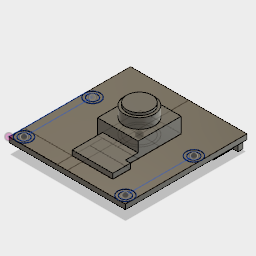
Pi Camera v2 (Autodesk Fusion 360 design; units mm, degrees)
Autodesk Fusion 360 part; units mm, degrees
sketch "Sketch1" plane through (0, 0, 0) normal (0, 1, 0) x (1, 0, 0)
  line L0 (0, 0) -> (23, 0)
  line L1 (23, 0) -> (23, 24)
  line L2 (23, 24) -> (0, 24)
  line L3 (0, 24) -> (0, 0)
  line L4 (0, 0) -> (9.4996, 0)
  line L5 (0, 3.5052) -> (0, 0)
  line L6 (0, 0) -> (9.5, 0)
  line L7 (0, 3) -> (0, 0)
  line L8 (9.5, 3) -> (17.5, 3)
  line L9 (17.5, 3) -> (17.5, 6.5)
  line L10 (17.5, 6.5) -> (9.5, 6.5)
  line L11 (9.5, 6.5) -> (9.5, 3)
  line L12 (9.5, 3) -> (0, 3)
  line L13 (9.5, 6.5) -> (16.5, 6.5)
  line L14 (16.5, 6.5) -> (16.5, 9)
  line L15 (16.5, 9) -> (9.5, 9)
  line L16 (9.5, 9) -> (9.5, 6.5)
  line L17 (16.5, 9) -> (7.5, 9)
  line L18 (7.5, 9) -> (7.5, 17.5)
  line L19 (7.5, 17.5) -> (16.5, 17.5)
  line L20 (16.5, 17.5) -> (16.5, 9)
  line L21 (12, 17.5) -> (12, 9)
  line L22 (7.5, 13.25) -> (16.5, 13.25)
  circle A0 centre (12, 13.25) radius 3.25
  circle A1 centre (12, 13.25) radius 2.5
  dimension "d1" = 23
  dimension "d2" = 24
  dimension "d22" = 9.5
  dimension "d23" = 3
  dimension "d25" = 3.5
  dimension "d28" = 7
  dimension "d29" = 2.5
  dimension "d30" = 8.5
  dimension "d31" = 9
  dimension "d32" = 6.5
  dimension "d33" = 5
  measures "d1" distance of L0.start L0.end
  measures "d2" distance of L0.start L2.end
  measures "d22" distance of L0.start L6.end
  measures "d23" distance of L0.start L7.start
  measures "d25" distance of L8.start L10.end
  measures "d28" distance of L10.end L13.end
  measures "d29" distance of L10.end L15.end
  measures "d30" distance of L14.end L19.end
  measures "d31" distance of L14.end L17.end
  measures "d32" diameter of A0
  measures "d33" diameter of A1
extrude "Extrude4" add sketch "Sketch1" along normal blind 1 contours L0 L1 L2 L3 L4 L5 L6 L7 | L8 L9 L10 L11 L13 | L10 L13 L14 L15 L16 L17 | L15 L17 L18 L21 L22 A0 | L15 L17 L20 L21 L22 A0 | L19 L20 L21 L22 A0 | L21 L22 A0 A1 | L21 L22 A0 A1 | L18 L19 L21 L22 A0 | L21 L22 A0 A1 | L21 L22 A1 | L21 L22 A1 | L21 L22 A0 A1 | L21 L22 A1 | L21 L22 A1 makes body 1
extrude "Extrude1" add sketch "Sketch1" along normal blind 1 separate body contours L0 L1 L2 L3 L4 L5 L6 L7 | L8 L9 L10 L11 L13 | L10 L13 L14 L15 L16 L17 | L15 L17 L18 L21 L22 A0 | L15 L17 L20 L21 L22 A0 | L19 L20 L21 L22 A0 | L21 L22 A0 A1 | L21 L22 A0 A1 | L18 L19 L21 L22 A0 | L21 L22 A0 A1 | L21 L22 A1 | L21 L22 A1 | L21 L22 A0 A1 | L21 L22 A1 | L21 L22 A1 makes body 2
sketch "Sketch2" plane through (0, 1, 0) normal (0, 1, 0) x (-1, 0, 0)
  line L0 (0, -24) -> (0, 0)
  line L1 (0, 0) -> (-23, 0)
  line L2 (-23, 0) -> (-23, -24)
  line L3 (-23, -24) -> (0, -24)
  line L4 (0, 0) -> (-9.5, 0)
  line L5 (-9.5, 0) -> (-9.5, -3)
  line L6 (-9.5, -3) -> (0, -3)
  line L7 (0, -3) -> (0, 0)
  line L8 (-9.5, -3) -> (-17.5, -3)
  line L9 (-17.5, -3) -> (-17.5, -6.5)
  line L10 (-17.5, -6.5) -> (-9.5, -6.5)
  line L11 (-9.5, -6.5) -> (-9.5, -3)
  line L12 (-9.5, -6.5) -> (-16.5, -6.5)
  line L13 (-16.5, -6.5) -> (-16.5, -9)
  line L14 (-16.5, -9) -> (-9.5, -9)
  line L15 (-9.5, -9) -> (-9.5, -6.5)
  line L16 (-16.5, -9) -> (-8.5, -9)
  line L17 (-8.5, -9) -> (-8.5, -17.5)
  line L18 (-8.5, -17.5) -> (-16.5, -17.5)
  line L19 (-16.5, -17.5) -> (-16.5, -9)
  line L20 (-12.5, -17.5) -> (-12.5, -9)
  line L21 (-8.5, -13.25) -> (-16.5, -13.25)
  circle A0 centre (-12.5, -13.25) radius 3
  circle A1 centre (-12.5, -13.25) radius 2.5
  line L22 (0, 0) -> (0, -15)
  line L23 (0, -15) -> (-1.5, -15)
  circle A2 centre (-1.5, -15) radius 1.5
  line L24 (-11.5, -24) -> (-11.5, 0)
  circle A3 centre (-21.5, -15) radius 1.5
  line L25 (-1.5, -15) -> (-1.5, -1.5)
  circle A4 centre (-1.5, -1.5) radius 1.4986
  line L26 (-21.5, -15) -> (-21.5, -1.5)
  circle A5 centre (-21.5, -1.5) radius 1.4986
  circle A6 centre (-1.5, -15) radius 1
  circle A7 centre (-1.5, -1.5) radius 1
  circle A8 centre (-21.5, -1.5) radius 1
  circle A9 centre (-21.5, -15) radius 1
  dimension "d36" = 9.5
  dimension "d37" = 3
  dimension "d38" = 3.5
  dimension "d39" = 8
  dimension "d40" = 7
  dimension "d41" = 2.5
  dimension "d42" = 8
  dimension "d43" = 8.5
  dimension "d44" = 6
  dimension "d45" = 5
  dimension "d58" = 15
  dimension "d59" = 1.5
  dimension "d61" = 13.5
  dimension "d62" = 2.9972
  dimension "d63" = 2.9972
  dimension "d64" = 2
  dimension "d65" = 2
  dimension "d66" = 2
  dimension "d67" = 2
  measures "d36" distance of L0.end L4.end
  measures "d37" distance of L0.end L6.end
  measures "d38" distance of L5.end L10.end
  measures "d39" distance of L5.end L8.end
  measures "d40" distance of L10.end L12.end
  measures "d41" distance of L10.end L14.end
  measures "d42" distance of L13.end L16.end
  measures "d43" distance of L13.end L18.end
  measures "d44" diameter of A0
  measures "d45" diameter of A1
  measures "d58" distance of L0.end L22.end
  measures "d59" distance of L22.end L23.end
  measures "d61" distance of L23.end L25.end
  measures "d62" diameter of A4
  measures "d63" diameter of A5
  measures "d64" diameter of A6
  measures "d65" diameter of A7
  measures "d66" diameter of A8
  measures "d67" diameter of A9
extrude "Extrude11" cut sketch "Sketch2" against normal blind 0.05 contours L23 A2 L25 A6 | L23 A2 L25 A6 | A4 | A3 | A5 bodies 2 1
extrude "Extrude7" add sketch "Sketch2" along normal blind 1 contours L8 L10 L11 L12 L24 | L8 L9 L10 L12 L24 | L10 L12 L14 L15 L16 L24 | L10 L12 L13 L14 L16 L24 bodies 2 1
extrude "Extrude8" add sketch "Sketch2" along normal blind 3 contours L17 L18 L21 A0 L24 | L18 L20 A0 L24 | L18 L19 L20 L21 A0 | L21 A0 A1 L24 | L20 A0 A1 L24 | L14 L16 L17 L21 A0 L24 | L20 L21 A0 A1 | L21 A0 A1 L24 | L21 A1 L24 | L20 L21 A1 L24 | L14 L16 L19 L20 L21 A0 | L20 L21 A1 | L20 L21 A0 A1 | L21 A1 L24 | L20 A0 A1 L24 | L14 L16 L20 A0 L24 | L20 L21 A1 L24 | L20 L21 A1 bodies 2
sketch "Sketch4" plane through (0, 4, 0) normal (0, 1, 0) x (-1, 0, 0)
  line L0 (-16.5, -17.5) -> (-8.5, -17.5)
  line L1 (-8.5, -17.5) -> (-8.5, -9)
  line L2 (-8.5, -9) -> (-16.5, -9)
  line L3 (-16.5, -9) -> (-16.5, -17.5)
  line L4 (-12.5, -17.5) -> (-12.5, -9)
  line L5 (-8.5, -13.25) -> (-16.5, -13.25)
  circle A0 centre (-12.5, -13.25) radius 3
  circle A1 centre (-12.5, -13.25) radius 3
  circle A2 centre (-12.5, -13.25) radius 2.5
  circle A3 centre (-12.5, -13.25) radius 2.5
  point P0 (-12.5, -17.5)
  point P1 (-12.5, -9)
  point P2 (-8.5, -13.25)
  point P3 (-16.5, -13.25)
  point P4 (-12.5, -13.25)
extrude "Extrude9" add sketch "Sketch4" along normal blind 2 contours L4 L5 A0 A1 A2 A3 | L4 L5 A0 A1 A2 A3 | L4 L5 A0 A1 A2 A3 | L4 L5 A2 A3 | L4 L5 A2 A3 | L4 L5 A0 A1 A2 A3 | L4 L5 A2 A3 | L4 L5 A2 A3 bodies 2
sketch "Sketch5" plane through (0, 6, 0) normal (0, 1, 0) x (-1, 0, 0)
  circle A0 centre (-12.5, -13.25) radius 3
  circle A1 centre (-12.5, -13.25) radius 2.5
  circle A2 centre (-12.5, -13.25) radius 2.5
extrude "Extrude10" add sketch "Sketch5" along normal blind 0.5 contours A1 A2 bodies 2
extrude "Extrude12" cut sketch "Sketch2" against normal through all contours L23 L25 A6 | L23 L25 A6 | A7 | A8 | A9 bodies 2
sketch "Sketch6" plane through (0, 0, 0) normal (0, -1, 0) x (1, 0, 0)
  circle A0 centre (21.5, -1.5) radius 1
  circle A1 centre (1.5, -1.5) radius 1
  circle A2 centre (21.5, -15) radius 1
  circle A3 centre (1.5, -15) radius 1
  line L0 (0, 0) -> (0, -24)
  line L1 (0, -24) -> (23, -24)
  line L2 (23, -24) -> (23, 0)
  line L3 (23, 0) -> (0, 0)
  line L4 (0, -24) -> (1, -24)
  line L5 (23, -24) -> (22.1897, -24)
  line L6 (22.1897, -24) -> (1, -24)
  line L7 (1, -24) -> (1, -23)
  line L8 (1, -23) -> (22.1897, -23)
  line L9 (22.1897, -23) -> (22.1897, -24)
  line L10 (22.1897, -23) -> (21.1897, -23)
  line L11 (21.1897, -23) -> (1.6897, -23)
  line L12 (1.6897, -23) -> (1.6897, -19)
  line L13 (1.6897, -19) -> (21.1897, -19)
  line L14 (21.1897, -19) -> (21.1897, -23)
  dimension "d71" = 1
  dimension "d72" = 0.8103
  dimension "d73" = 1
  dimension "d74" = 1
  dimension "d75" = 19.5
  dimension "d76" = 4
  measures "d71" distance of L0.end L4.end
  measures "d72" distance of L1.end L5.end
  measures "d73" distance of L5.end L8.end
  measures "d74" distance of L8.end L10.end
  measures "d75" distance of L10.end L11.end
  measures "d76" distance of L10.end L13.end
extrude "Extrude13" add sketch "Sketch6" along normal blind 2 separate body contours L1 L6 L7 L8 L9 L10 L11 | L8 L11 L12 L13 L14 makes body 3
